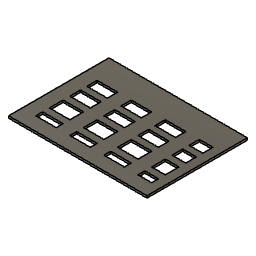
keypad+spacer (Autodesk Fusion 360 design; units mm, degrees)
Autodesk Fusion 360 part; units mm, degrees
sketch "Sketch1" plane through (0, 0, 0) normal (0, 0, 1) x (1, 0, 0)
  line L0 (0, 0) -> (101.6, 0)
  line L1 (101.6, 0) -> (101.6, 73.66)
  line L2 (101.6, 73.66) -> (0, 73.66)
  line L3 (0, 73.66) -> (0, 0)
  dimension "d1" = 101.6
  dimension "d2" = 73.66
  constraint coincident L0.start L3.end
  constraint horizontal L0
  constraint perpendicular L0 L1
  constraint perpendicular L1 L2
  constraint perpendicular L0 L3
  measures "d1" distance of L0.start L0.end
  measures "d2" distance of L0.end L1.end
extrude "Extrude1" add sketch "Sketch1" along normal blind 1.5
sketch "Sketch2" plane through (0, 0, 1.5) normal (0, 0, 1) x (-1, 0, 0)
  line L0 (0, -73.66) -> (0, 0)
  line L1 (0, 0) -> (-101.6, 0)
  line L2 (-101.6, 0) -> (-101.6, -73.66)
  line L3 (-101.6, -73.66) -> (0, -73.66)
  line L4 (-10, -35) -> (-25, -35)
  line L5 (-10, -30) -> (-25, -30)
  line L6 (-35, -35) -> (-50, -35)
  line L7 (-35, -30) -> (-50, -30)
  line L8 (-60, -35) -> (-75, -35)
  line L9 (-85, -35) -> (-95, -35)
  line L10 (-60, -30) -> (-75, -30)
  line L11 (-85, -30) -> (-95, -30)
  line L12 (-25, -55) -> (-10, -55)
  line L13 (-50, -55) -> (-35, -55)
  line L14 (-95, -55) -> (-85, -55)
  line L15 (-75, -55) -> (-60, -55)
  line L16 (-85, -10) -> (-95, -10)
  line L17 (-60, -10) -> (-75, -10)
  line L18 (-10, -10) -> (-25, -10)
  line L19 (-35, -10) -> (-50, -10)
  line L20 (-10, -20) -> (-95, -20)
  line L21 (-10, -15) -> (-95, -15)
  line L22 (-25, -30) -> (-25, -20)
  line L23 (-25, -15) -> (-25, -10)
  line L24 (-10, -10) -> (-10, -15)
  line L25 (-10, -20) -> (-10, -30)
  line L26 (-35, -30) -> (-35, -20)
  line L27 (-35, -15) -> (-35, -10)
  line L28 (-50, -30) -> (-50, -20)
  line L29 (-50, -15) -> (-50, -10)
  line L30 (-60, -30) -> (-60, -20)
  line L31 (-60, -15) -> (-60, -10)
  line L32 (-75, -30) -> (-75, -20)
  line L33 (-75, -15) -> (-75, -10)
  line L34 (-85, -30) -> (-85, -20)
  line L35 (-85, -15) -> (-85, -10)
  line L36 (-95, -30) -> (-95, -20)
  line L37 (-95, -15) -> (-95, -10)
  line L38 (-10, -35) -> (-10, -42.8011)
  line L39 (-10, -47.4728) -> (-10, -55)
  line L40 (-25, -55) -> (-25, -47.4728)
  line L41 (-25, -42.8011) -> (-25, -35)
  line L42 (-35, -55) -> (-35, -47.4728)
  line L43 (-35, -42.8011) -> (-35, -35)
  line L44 (-10, -42.8011) -> (-25, -42.8011)
  line L45 (-10, -47.4728) -> (-25, -47.4728)
  line L46 (-35, -47.4728) -> (-50, -47.4728)
  line L47 (-35, -42.8011) -> (-50, -42.8011)
  line L48 (-50, -55) -> (-50, -47.4728)
  line L49 (-50, -42.8011) -> (-50, -35)
  line L50 (-60, -55) -> (-60, -47.4728)
  line L51 (-60, -42.8011) -> (-60, -35)
  line L52 (-60, -47.4728) -> (-75, -47.4728)
  line L53 (-85, -47.4728) -> (-95, -47.4728)
  line L54 (-75, -55) -> (-75, -47.4728)
  line L55 (-75, -42.8011) -> (-75, -35)
  line L56 (-60, -42.8011) -> (-75, -42.8011)
  line L57 (-85, -42.8011) -> (-95, -42.8011)
  line L58 (-85, -55) -> (-85, -47.4728)
  line L59 (-85, -42.8011) -> (-85, -35)
  line L60 (-95, -55) -> (-95, -47.4728)
  line L61 (-95, -42.8011) -> (-95, -35)
  constraint coincident L4.start L24
  constraint perpendicular L4 L60
  constraint coincident L11.end L60
  constraint perpendicular L5 L60
  constraint collinear L22 L40
  constraint coincident L6.start L4
  constraint coincident L7.start L5
  constraint collinear L26 L42
  constraint collinear L4 L6
  constraint collinear L5 L7
  constraint collinear L6 L8
  constraint coincident L7.end L48
  constraint coincident L10.start L50
  constraint collinear L7 L10
  constraint collinear L28 L48
  constraint collinear L30 L50
  constraint collinear L24 L38
  constraint collinear L8 L9
  constraint coincident L10.end L54
  constraint coincident L11.start L58
  constraint collinear L10 L11
  constraint collinear L32 L54
  constraint collinear L34 L58
  constraint collinear L36 L60
  constraint perpendicular L18 L36
  constraint perpendicular L14 L38
  constraint coincident L12.start L14
  constraint coincident L13.start L14
  constraint coincident L15.start L14
  constraint collinear L12 L14
  constraint collinear L13 L14
  constraint collinear L14 L15
  constraint collinear L16 L18
  constraint coincident L17.start L18
  constraint collinear L17 L18
  constraint coincident L19.start L18
  constraint collinear L18 L19
  constraint coincident L21.end L36
  constraint perpendicular L21 L36
  constraint coincident L20 L22.end
  constraint coincident L21 L23.start
  constraint collinear L22 L23
  constraint collinear L24 L25
  constraint coincident L20.start L24
  constraint coincident L20 L26.end
  constraint coincident L21 L27.start
  constraint collinear L26 L27
  constraint coincident L20 L28.end
  constraint coincident L21 L29.start
  constraint collinear L28 L29
  constraint coincident L20 L30.end
  constraint coincident L21 L31.start
  constraint collinear L30 L31
  constraint coincident L20 L32.end
  constraint coincident L21 L33.start
  constraint collinear L32 L33
  constraint coincident L20 L34.end
  constraint coincident L21 L35.start
  constraint collinear L34 L35
  constraint collinear L36 L37
  constraint coincident L39.start L38
  constraint perpendicular L45 L60
  constraint coincident L57.end L60
  constraint perpendicular L44 L60
  constraint collinear L38 L39
  constraint collinear L40 L41
  constraint coincident L42.end L45
  constraint coincident L43.start L44
  constraint collinear L42 L43
  constraint collinear L44 L47
  constraint collinear L45 L46
  constraint collinear L46 L52
  constraint coincident L47.end L48
  constraint coincident L51.start L50
  constraint collinear L47 L56
  constraint collinear L48 L49
  constraint collinear L50 L51
  constraint collinear L52 L53
  constraint collinear L54 L55
  constraint coincident L57.start L58
  constraint collinear L56 L57
  constraint collinear L58 L59
  constraint collinear L60 L61
extrude "Extrude2" cut sketch "Sketch2" against normal blind 5 contours L4 L38 L41 L44 | L5 L20 L22 L25 | L6 L43 L47 L49 | L7 L20 L26 L28 | L8 L51 L55 L56 | L9 L57 L59 L61 | L10 L20 L30 L32 | L11 L20 L34 L36 | L12 L39 L40 L45 | L13 L42 L46 L48 | L14 L53 L58 L60 | L15 L50 L52 L54 | L16 L21 L35 L37 | L17 L21 L31 L33 | L18 L21 L23 L24 | L19 L21 L27 L29
